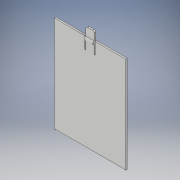
# Autodesk Inventor part: BatteryBoxLid
Saved by Autodesk Inventor 2019 (Build 230136000, 136)
## iProperties
Created: 2018-06-02
Part Number: BatteryBoxLid
Material: Generic
Document SubType Name: Modeling
Designer: samps
Density: 1 g/cm^3
Appearance: Default
Author: samps
Autodesk Inventor part; units mm, degrees
ref_plane "YZ Plane" through (0, 0, 0) normal (1, 0, 0) x (0, 1, 0)
ref_plane "XZ Plane" through (0, 0, 0) normal (0, 1, 0) x (-1, 0, 0)
ref_plane "XY Plane" through (0, 0, 0) normal (0, 0, 1) x (1, 0, 0)
sketch "Sketch1" plane through (0, 0, 0) normal (0, 0, 1) x (1, 0, 0)
  line L0 (0, 0) -> (85.5, 0)
  line L1 (85.5, 0) -> (85.5, -116.825)
  line L2 (85.5, -116.825) -> (0, -116.825)
  line L3 (0, -116.825) -> (0, 0)
  dimension "d0" = 85.5
  dimension "d1" = 116.825
  constraints: 8 end point, 2 parallel, 1 horizontal, 1 perpendicular
  measures "d0" distance of L1.end L2.end
  measures "d1" distance of L0.end L1.end
extrude "Extrusion1" add sketch "Sketch1" along normal blind 2
sketch "Sketch2" plane through (0, 0, 0) normal (0, 0, -1) x (-1, 0, 0)
  line L0 (-85.5, 0) -> (0, 0) projected
  line L1 (0, 0) -> (-42.75, 0)
  line L2 (-42.75, 0) -> (-47.75, 0)
  line L3 (-47.75, 0) -> (-37.75, 0)
  line L4 (-37.75, 0) -> (-37.75, 10)
  line L5 (-37.75, 10) -> (-47.75, 10)
  line L6 (-47.75, 10) -> (-47.75, 0)
  dimension "d4" = 5
  dimension "d5" = 10
  dimension "d6" = 10
  constraints: 12 end point, 2 parallel, 1 horizontal, 1 midpoint, 1 perpendicular, 1 point on line
  measures "d4" distance of L1.end L2.end
  measures "d5" distance of L5.end L4.end
  measures "d6" distance of L4.end L3.end
extrude "Extrusion2" add sketch "Sketch2" against normal blind 2
sketch "Sketch3" plane through (0, 0, 2) normal (0, 0, 1) x (1, 0, 0)
  line L0 (0, 0) -> (37.75, 0) projected
  line L1 (37.75, 0) -> (37.75, -13.175)
  line L2 (37.75, -13.175) -> (47.75, -13.175)
  line L3 (47.75, 0) -> (47.75, 10) projected
  line L4 (47.75, -13.175) -> (47.75, 0)
  line L5 (47.75, 0) -> (48.75, 0)
  line L6 (47.75, 0) -> (85.5, 0) projected
  line L7 (48.75, 0) -> (48.75, -13.175)
  line L8 (48.75, -13.175) -> (48.75, -14.175)
  line L9 (48.75, -14.175) -> (37.75, -14.175)
  line L10 (37.75, -14.175) -> (36.75, -14.175)
  line L11 (36.75, -14.175) -> (36.75, 0)
  line L12 (37.75, -13.175) -> (37.75, -14.175)
  line L13 (47.75, -13.175) -> (47.75, -14.175)
  dimension "d9" = 13.175
  dimension "d10" = 1
  dimension "d11" = 1
  dimension "d12" = 1
  constraints: 22 end point, 7 point on line, 6 perpendicular, 1 parallel, 1 vertical
  measures "d9" distance of L0.end L1.end
  measures "d10" distance of L3.start L5.end
  measures "d11" distance of L7.end L8.end
  measures "d12" distance of L9.end L10.end
extrude "Extrusion3" cut sketch "Sketch3" against normal blind 3.175 contours L0 L1 L12 L10 L11 | L4 L5 L7 L8 L9 L13
sketch "Sketch4" plane through (0, 0, 2) normal (0, 0, 1) x (1, 0, 0)
  line L0 (37.75, 10) -> (37.75, -14.175) projected
  line L1 (47.75, -14.175) -> (47.75, 10) projected
  line L2 (37.75, 0) -> (47.75, 0)
  line L3 (47.75, 0) -> (47.75, -4)
  line L4 (47.75, -4) -> (37.75, -4)
  line L5 (37.75, -4) -> (37.75, 0)
  point P0 (0, 0)
  dimension "d15" = 4
  constraints: 8 end point, 2 parallel, 2 point on line, 1 horizontal, 1 perpendicular
  measures "d15" distance of L2.end L3.end
extrude "Extrusion4" add sketch "Sketch4" along normal blind 2
fillet "Fillet1" radius 2 2 edges at (42.75, 0, 4) (42.75, -4, 4)
fillet "Fillet2" radius 2 3 edges at (0, -116.825, 1) (85.5, -116.825, 1) (42.75, -116.825, 2)
fillet "Fillet3" radius 2 2 edges at (37.75, 10, 1) (47.75, 10, 1)
body "Solid1"
